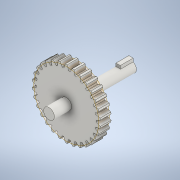
# Autodesk Inventor part: Spur Gear2
Saved by Autodesk Inventor 2021 (Build 250183000, 183)
## iProperties
Created: 2021-04-10
Part Number: Spur Gear2
Material: Steel
Document SubType Name: Modeling
Designer: Nabeel Azafer
Categories: <?xml version="1.0" encoding="UTF-16"?> <MemberInstance><Categories><FamilyTemplate><FamilyTemplateParameter ValueType="xs:double" Id="1" ObjectReferenceKey="da_z" ObjectType="kUserParameterObject"/><FamilyTemplateParameter ValueType="xs:double" Id="2" ObjectReferenceKey="da_b" ObjectType="kUserParameterObject"/><FamilyTemplateParameter ValueType="xs:double" Id="3" ObjectReferenceKey="da_beta" ObjectType="kUserParameterObject"/><FamilyTemplateParameter ValueType="xs:double" Id="4" ObjectReferenceKey="da_da" ObjectType="kUserParameterObject"/><FamilyTemplateParameter ValueType="xs:double" Id="5" ObjectReferenceKey="da_aw" ObjectType="kUserParameterObject"/><FamilyTemplateParameter ValueType="xs:string" Id="6" ObjectReferenceKey="EAIAABAAAACIAQAAAAAAAIAAAAAAAAAA" ObjectType="83910656" SubObjectId="SurfaceGeometry"/></FamilyTemplate><ParamToTemplateMap><ParamToTemplate CategoryParameter="//CategoryParameter[@InternalName='046C89C9-8512-4d59-83FE-43B91F4F132A']" TemplateParameter="1"/><ParamToTemplate CategoryParameter="//CategoryParameter[@InternalName='2552DF32-E462-4b46-AEBF-C6C7768E72AC']" TemplateParameter="2"/><ParamToTemplate CategoryParameter="//CategoryParameter[@InternalName='C9EE641D-15FC-4fae-A226-E94C4372FDD7']" TemplateParameter="3"/><ParamToTemplate><ParamToTemplate CategoryParameter="//CategoryParameter[@InternalName='00B6519A-459B-49c7-AD84-2E56D39A5744']" ConstantValue="0.000000"/></ParamToTemplate><ParamToTemplate><ParamToTemplate CategoryParameter="//CategoryParameter[@InternalName='04B31F0E-C7A6-4894-AA32-9629BEFACF47']" ConstantValue="0.800000"/></ParamToTemplate><ParamToTemplate><ParamToTemplate CategoryParameter="//CategoryParameter[@InternalName='43CBEC2E-7847-49e7-A936-2F7889FCB2D9']" ConstantValue="0.350000"/></ParamToTemplate><ParamToTemplate><ParamToTemplate CategoryParameter="//CategoryParameter[@InternalName='B1EFC894-105D-4ebd-86BF-FA20ED196853']" ConstantValue="0.500000"/></ParamToTemplate><ParamToTemplate><ParamToTemplate CategoryParameter="//CategoryParameter[@InternalName='51175063-3D10-4879-93E8-6246FE8B403D']" ConstantValue="2060000000.000000"/></ParamToTemplate><ParamToTemplate><ParamToTemplate CategoryParameter="//CategoryParameter[@InternalName='A3A52E27-4454-46a9-B0BD-C932399B70AF']" ConstantValue="0.300000"/></ParamToTemplate><ParamToTemplate><ParamToTemplate CategoryParameter="//CategoryParameter[@InternalName='91B76062-C214-41d9-B1B9-14D2AB99603D']" ConstantValue="0.100000"/></ParamToTemplate><ParamToTemplate><ParamToTemplate CategoryParameter="//CategoryParameter[@InternalName='374E806E-8B8A-4dda-A9AA-1039D6500AD2']" ConstantValue="10.000000"/></ParamToTemplate><ParamToTemplate><ParamToTemplate CategoryParameter="//CategoryParameter[@InternalName='2D373A89-B862-43d6-8D0B-0CBF12AB9F6C']" ConstantValue="0.349066"/></ParamToTemplate><ParamToTemplate CategoryParameter="//CategoryParameter[@InternalName='37777632-D6A2-4fac-9D53-DB8ACD95C989']" TemplateParameter="4"/><ParamToTemplate CategoryParameter="//CategoryParameter[@InternalName='FD1017F1-B727-4f7e-9707-0F86F1FF9423']" TemplateParameter="5"/><ParamToTemplate><ParamToTemplate CategoryParameter="//CategoryParameter[@InternalName='9E1B4470-B2D3-4ff1-B813-535BB4CDF51A']" ConstantValue="3520000.000000"/></ParamToTemplate><ParamToTemplate><ParamToTemplate CategoryParameter="//CategoryParameter[@InternalName='F8452263-BFF6-458c-9FB1-07C4B99E95CD']" ConstantValue="11400000.000000"/></ParamToTemplate><ParamToTemplate><ParamToTemplate CategoryParameter="//CategoryParameter[@InternalName='3E3BB259-FD49-497f-8171-6EBC954A3479']" ConstantValue="2.000000"/></ParamToTemplate><ParamToTemplate CategoryParameter="//CategoryParameter[@InternalName='27C3BAF2-7550-4e4b-AE2C-0DB134B7D9B7']" TemplateParameter="6"/></ParamToTemplateMap><Category DisplayName="Gear" InternalName="DC85795E-93AB-48d5-8EEE-5A27447B64BD" Mnemonic="Gear"><CategoryParameter DisplayName="z" InternalName="046C89C9-8512-4d59-83FE-43B91F4F132A" Mnemonic="z"/><CategoryParameter DisplayName="b" InternalName="2552DF32-E462-4b46-AEBF-C6C7768E72AC" Mnemonic="b"/><CategoryParameter DisplayName="||b|" InternalName="C9EE641D-15FC-4fae-A226-E94C4372FDD7" Mnemonic="beta"/><CategoryParameter DisplayName="x" InternalName="00B6519A-459B-49c7-AD84-2E56D39A5744" Mnemonic="x"/><CategoryParameter DisplayName="a*" InternalName="04B31F0E-C7A6-4894-AA32-9629BEFACF47" Mnemonic="a"/><CategoryParameter DisplayName="c*" InternalName="43CBEC2E-7847-49e7-A936-2F7889FCB2D9" Mnemonic="c"/><CategoryParameter DisplayName="r|.f|*" InternalName="B1EFC894-105D-4ebd-86BF-FA20ED196853" Mnemonic="rf"/><CategoryParameter DisplayName="E" InternalName="51175063-3D10-4879-93E8-6246FE8B403D" Mnemonic="E"/><CategoryParameter DisplayName="||m|" InternalName="A3A52E27-4454-46a9-B0BD-C932399B70AF" Mnemonic="mi"/><Category DisplayName="SpurGear" InternalName="26C5A22E-A91E-4dfd-A3B3-23CCAFAE1764" Mnemonic="SpurGear"><CategoryParameter DisplayName="m" InternalName="91B76062-C214-41d9-B1B9-14D2AB99603D" Mnemonic="m"/><CategoryParameter DisplayName="P" InternalName="374E806E-8B8A-4dda-A9AA-1039D6500AD2" Mnemonic="PP"/><CategoryParameter DisplayName="||a|" InternalName="2D373A89-B862-43d6-8D0B-0CBF12AB9F6C" Mnemonic="alpha"/><CategoryParameter DisplayName="d|.a|" InternalName="37777632-D6A2-4fac-9D53-DB8ACD95C989" Mnemonic="da"/><CategoryParameter DisplayName="a|.w|" InternalName="FD1017F1-B727-4f7e-9707-0F86F1FF9423" Mnemonic="aw"/><CategoryParameter DisplayName="||s||.Flim|" InternalName="9E1B4470-B2D3-4ff1-B813-535BB4CDF51A" Mnemonic="sFlim"/><CategoryParameter DisplayName="||s||.Hlim|" InternalName="F8452263-BFF6-458c-9FB1-07C4B99E95CD" Mnemonic="sHlim"/><CategoryParameter DisplayName="type" InternalName="3E3BB259-FD49-497f-8171-6EBC954A3479" Mnemonic="type"/><CategoryParameter DisplayName="PitchDiameter" InternalName="27C3BAF2-7550-4e4b-AE2C-0DB134B7D9B7" Mnemonic="IDS_PITCHDIAM"/></Category></Category></Categories></MemberInstance>
Density: 7.85 g/cm^3
Appearance: Steel
Mass: 43.2565 g
Surface Area: 28.3538 cm^2
Volume: 5.51038 cm^3
Author: Nabeel Azafer
Autodesk Inventor part; units mm, degrees
note: some values were not read from the file. Chosen so that the rebuilt part matches the saved one: direction of "Emboss1".
sketch "Sketch1" plane through (0, 0, 0) normal (0, 0, 1) x (1, 0, 0)
  circle A0 centre (0, 0) radius 15.8
  dimension "d0" = 31.6
  constraints: 1 centre point
  measures "d0" diameter of A0
extrude "Extrusion1" add sketch "Sketch1" along normal blind 5
ref_plane "Work Plane2" through (0, 0, 2.5) normal (0, 0, 1) x (1, 0, 0)
sketch "Sketch2" plane through (0, 0, 0) normal (0, 0, -1) x (-1, 0, 0)
  circle A0 centre (0, 0) radius 15.8 projected
  circle A1 centre (0, 0) radius 15
  dimension "d3" = 30
  constraints: 1 centre point, 1 coincident
  measures "d3" diameter of A1
surface extrude "Pitch Diameter" sketch "Sketch2" against normal through all shown yes curves A1
ref_plane "Work Plane8" through (0, 0, 0) normal (0.9945219, 0.1045285, 0) x (0, 0, 1)
ref_plane "Work Plane9" through (0, 0, 0) normal (1, 0, 0) x (0, 1, 0)
spur gear teeth "Spur Gear" teeth 30 pitch diameter 30 tip diameter 31.6 root diameter 27.7 face width 8 start plane through (0, 0, 0) normal (0, 0, -1) x (-1, 0, 0)
sketch "Sketch6" plane through (0, 0, 0) normal (0, 0, -1) x (-1, 0, 0)
  circle A0 centre (0, 0) radius 2.5
  dimension "d68" = 5
  constraints: 1 centre point, 1 coincident
  measures "d68" diameter of A0
extrude "Extrusion4" add sketch "Sketch6" along normal blind 25
sketch "Sketch7" plane through (0, 0, -25) normal (0, 0, -1) x (-1, 0, 0)
  circle A0 centre (0, 0) radius 2.5 projected
  line L0 (-1, 2.2913) -> (1, 2.2913)
  line L1 (1, 2.2913) -> (1, 3.7913)
  line L2 (1, 3.7913) -> (-1, 3.7913)
  line L3 (-1, 3.7913) -> (-1, 2.2913)
  dimension "d75" = 2
  dimension "d76" = 1.5
  constraints: 8 end point, 2 parallel, 1 horizontal, 1 perpendicular, 2 other
  measures "d75" distance of L2.end L1.end
  measures "d76" distance of L1.end L0.end
extrude "Extrusion5" add sketch "Sketch7" against normal blind 6 contours L0 A0 | A0 L3 L2 L1 picked at (-0.1703, 2.3433)
sketch "Sketch8" plane through (0, 0, 5) normal (0, 0, 1) x (1, 0, 0)
  circle A0 centre (0, 0) radius 2.5
  dimension "d79" = 5
  constraints: 1 centre point, 1 coincident
  measures "d79" diameter of A0
extrude "Extrusion6" add sketch "Sketch8" along normal blind 8
sketch "Sketch9" plane through (0, 0, 0) normal (0, 0, -1) x (-1, 0, 0)
  line L0 (-6.4513, 9.2943) -> (6.8887, 9.2943) construction
  line L1 (6.8887, 9.2943) -> (6.8887, 2.6243) construction
  line L2 (6.8887, 2.6243) -> (-6.4513, 2.6243) construction
  line L3 (-6.4513, 2.6243) -> (-6.4513, 9.2943) construction
  spline S0 degree 2 poles (-5.4108, 7.2132) (-5.6231, 7.2132) (-5.9748, 7.3429) (-6.1012, 7.4742) knots 0 0 0 1 2 2 2
  spline S1 degree 2 poles (-6.1012, 7.4742) (-6.2277, 7.6071) (-6.3622, 7.9993) (-6.3622, 8.2538) knots 0 0 0 1 2 2 2
  spline S2 degree 2 poles (-6.3622, 8.2538) (-6.3622, 8.4953) (-6.226, 8.8777) (-6.0996, 9.0139) knots 0 0 0 1 2 2 2
  spline S3 degree 2 poles (-6.0996, 9.0139) (-5.9781, 9.1452) (-5.6215, 9.2878) (-5.4092, 9.2878) knots 0 0 0 1 2 2 2
  spline S4 degree 2 poles (-5.4092, 9.2878) (-5.3071, 9.2878) (-5.1223, 9.2586) (-5.038, 9.2327) knots 0 0 0 1 2 2 2
  spline S5 degree 2 poles (-5.038, 9.2327) (-4.97, 9.2132) (-4.8046, 9.1419) (-4.7544, 9.116) knots 0 0 0 1 2 2 2
  line L4 (-4.7544, 9.116) -> (-4.7544, 8.7951)
  line L5 (-4.7544, 8.7951) -> (-4.7771, 8.7951)
  spline S6 degree 2 poles (-4.7771, 8.7951) (-4.8273, 8.8389) (-4.9327, 8.9183) (-5.0299, 8.9636) knots 0 0 0 1 2 2 2
  spline S7 degree 2 poles (-5.0299, 8.9636) (-5.111, 9.0042) (-5.32, 9.0577) (-5.44, 9.0577) knots 0 0 0 1 2 2 2
  spline S8 degree 2 poles (-5.44, 9.0577) (-5.7285, 9.0577) (-6.085, 8.6233) (-6.085, 8.2619) knots 0 0 0 1 2 2 2
  spline S9 degree 2 poles (-6.085, 8.2619) (-6.085, 8.0609) (-5.991, 7.7594) (-5.9019, 7.6557) knots 0 0 0 1 2 2 2
  spline S10 degree 2 poles (-5.9019, 7.6557) (-5.816, 7.552) (-5.5729, 7.4434) (-5.4205, 7.4434) knots 0 0 0 1 2 2 2
  spline S11 degree 2 poles (-5.4205, 7.4434) (-5.3087, 7.4434) (-5.085, 7.4758) (-5.0089, 7.5082) knots 0 0 0 1 2 2 2
  line L6 (-5.0089, 7.5082) -> (-5.0089, 8.0252)
  line L7 (-5.0089, 8.0252) -> (-5.4724, 8.0252)
  line L8 (-5.4724, 8.0252) -> (-5.4724, 8.2586)
  line L9 (-5.4724, 8.2586) -> (-4.7463, 8.2586)
  line L10 (-4.7463, 8.2586) -> (-4.7463, 7.385)
  spline S12 degree 2 poles (-4.7463, 7.385) (-4.7965, 7.3624) (-4.9683, 7.2927) (-5.0413, 7.2716) knots 0 0 0 1 2 2 2
  spline S13 degree 2 poles (-5.0413, 7.2716) (-5.1401, 7.2424) (-5.299, 7.2132) (-5.4108, 7.2132) knots 0 0 0 1 2 2 2
  spline S14 degree 2 poles (-3.7803, 7.2181) (-4.1401, 7.2181) (-4.5356, 7.6217) (-4.5356, 7.9944) knots 0 0 0 1 2 2 2
  spline S15 degree 2 poles (-4.5356, 7.9944) (-4.5356, 8.3607) (-4.1515, 8.7951) (-3.8419, 8.7951) knots 0 0 0 1 2 2 2
  spline S16 degree 2 poles (-3.8419, 8.7951) (-3.7025, 8.7951) (-3.487, 8.7141) (-3.4076, 8.6282) knots 0 0 0 1 2 2 2
  spline S17 degree 2 poles (-3.4076, 8.6282) (-3.3265, 8.5423) (-3.2406, 8.2943) (-3.2406, 8.1144) knots 0 0 0 1 2 2 2
  line L11 (-3.2406, 8.1144) -> (-3.2406, 7.9766)
  line L12 (-3.2406, 7.9766) -> (-4.2795, 7.9766)
  spline S18 degree 2 poles (-4.2795, 7.9766) (-4.2795, 7.7157) (-4.017, 7.4385) (-3.7836, 7.4385) knots 0 0 0 1 2 2 2
  spline S19 degree 2 poles (-3.7836, 7.4385) (-3.7009, 7.4385) (-3.5405, 7.4758) (-3.4756, 7.505) knots 0 0 0 1 2 2 2
  spline S20 degree 2 poles (-3.4756, 7.505) (-3.4076, 7.5374) (-3.3136, 7.5941) (-3.2828, 7.6201) knots 0 0 0 1 2 2 2
  line L13 (-3.2828, 7.6201) -> (-3.2682, 7.6201)
  line L14 (-3.2682, 7.6201) -> (-3.2682, 7.3445)
  spline S21 degree 2 poles (-3.2682, 7.3445) (-3.3119, 7.3267) (-3.4448, 7.2748) (-3.4967, 7.2602) knots 0 0 0 1 2 2 2
  spline S22 degree 2 poles (-3.4967, 7.2602) (-3.5696, 7.2392) (-3.6896, 7.2181) (-3.7803, 7.2181) knots 0 0 0 1 2 2 2
  spline S23 degree 2 poles (-3.487, 8.1695) (-3.4902, 8.2716) (-3.5324, 8.4207) (-3.5729, 8.4709) knots 0 0 0 1 2 2 2
  spline S24 degree 2 poles (-3.5729, 8.4709) (-3.6166, 8.5277) (-3.7544, 8.5876) (-3.8565, 8.5876) knots 0 0 0 1 2 2 2
  spline S25 degree 2 poles (-3.8565, 8.5876) (-3.957, 8.5876) (-4.098, 8.5277) (-4.1563, 8.4693) knots 0 0 0 1 2 2 2
  spline S26 degree 2 poles (-4.1563, 8.4693) (-4.2131, 8.4094) (-4.2714, 8.2651) (-4.2795, 8.1695) knots 0 0 0 1 2 2 2
  line L15 (-4.2795, 8.1695) -> (-3.487, 8.1695)
  spline S27 degree 2 poles (-2.1482, 7.411) (-2.179, 7.3883) (-2.2828, 7.3072) (-2.3314, 7.2829) knots 0 0 0 1 2 2 2
  spline S28 degree 2 poles (-2.3314, 7.2829) (-2.3978, 7.2473) (-2.5226, 7.21) (-2.6361, 7.21) knots 0 0 0 1 2 2 2
  spline S29 degree 2 poles (-2.6361, 7.21) (-2.7285, 7.21) (-2.8954, 7.2797) (-2.9586, 7.3429) knots 0 0 0 1 2 2 2
  spline S30 degree 2 poles (-2.9586, 7.3429) (-3.0186, 7.4045) (-3.0915, 7.586) (-3.0915, 7.6865) knots 0 0 0 1 2 2 2
  spline S31 degree 2 poles (-3.0915, 7.6865) (-3.0915, 7.8421) (-2.9602, 8.0625) (-2.8176, 8.1257) knots 0 0 0 1 2 2 2
  spline S32 degree 2 poles (-2.8176, 8.1257) (-2.6912, 8.1841) (-2.3476, 8.2278) (-2.1482, 8.2392) knots 0 0 0 1 2 2 2
  line L16 (-2.1482, 8.2392) -> (-2.1482, 8.2878)
  spline S33 degree 2 poles (-2.1482, 8.2878) (-2.1482, 8.3753) (-2.2017, 8.4839) (-2.2504, 8.5147) knots 0 0 0 1 2 2 2
  spline S34 degree 2 poles (-2.2504, 8.5147) (-2.299, 8.5455) (-2.4384, 8.5649) (-2.5129, 8.5649) knots 0 0 0 1 2 2 2
  spline S35 degree 2 poles (-2.5129, 8.5649) (-2.6004, 8.5649) (-2.8371, 8.5131) (-2.9554, 8.4628) knots 0 0 0 1 2 2 2
  line L17 (-2.9554, 8.4628) -> (-2.97, 8.4628)
  line L18 (-2.97, 8.4628) -> (-2.97, 8.7205)
  spline S36 degree 2 poles (-2.97, 8.7205) (-2.9003, 8.74) (-2.6393, 8.7886) (-2.5113, 8.7886) knots 0 0 0 1 2 2 2
  spline S37 degree 2 poles (-2.5113, 8.7886) (-2.3557, 8.7886) (-2.1434, 8.74) (-2.0591, 8.6768) knots 0 0 0 1 2 2 2
  spline S38 degree 2 poles (-2.0591, 8.6768) (-1.9764, 8.6152) (-1.8954, 8.4191) (-1.8954, 8.2781) knots 0 0 0 1 2 2 2
  line L19 (-1.8954, 8.2781) -> (-1.8954, 7.2521)
  line L20 (-1.8954, 7.2521) -> (-2.1482, 7.2521)
  line L21 (-2.1482, 7.2521) -> (-2.1482, 7.411)
  line L22 (-2.1482, 7.6217) -> (-2.1482, 8.0382)
  spline S39 degree 2 poles (-2.1482, 8.0382) (-2.239, 8.0301) (-2.5129, 8.0025) (-2.5988, 7.9766) knots 0 0 0 1 2 2 2
  spline S40 degree 2 poles (-2.5988, 7.9766) (-2.6993, 7.9458) (-2.8306, 7.8178) (-2.8306, 7.7043) knots 0 0 0 1 2 2 2
  spline S41 degree 2 poles (-2.8306, 7.7043) (-2.8306, 7.5747) (-2.6847, 7.4434) (-2.5453, 7.4434) knots 0 0 0 1 2 2 2
  spline S42 degree 2 poles (-2.5453, 7.4434) (-2.427, 7.4434) (-2.2325, 7.5455) (-2.1482, 7.6217) knots 0 0 0 1 2 2 2
  line L23 (-0.7447, 8.4823) -> (-0.7576, 8.4823)
  spline S43 degree 2 poles (-0.7576, 8.4823) (-0.7868, 8.4904) (-0.85, 8.4936) (-0.8938, 8.4936) knots 0 0 0 1 2 2 2
  spline S44 degree 2 poles (-0.8938, 8.4936) (-0.9959, 8.4936) (-1.1969, 8.4045) (-1.2876, 8.317) knots 0 0 0 1 2 2 2
  line L24 (-1.2876, 8.317) -> (-1.2876, 7.2521)
  line L25 (-1.2876, 7.2521) -> (-1.5405, 7.2521)
  line L26 (-1.5405, 7.2521) -> (-1.5405, 8.753)
  line L27 (-1.5405, 8.753) -> (-1.2876, 8.753)
  line L28 (-1.2876, 8.753) -> (-1.2876, 8.5293)
  spline S45 degree 2 poles (-1.2876, 8.5293) (-1.1499, 8.6525) (-0.944, 8.753) (-0.8468, 8.753) knots 0 0 0 1 2 2 2
  spline S46 degree 2 poles (-0.8468, 8.753) (-0.8079, 8.753) (-0.769, 8.7497) (-0.7447, 8.7448) knots 0 0 0 1 2 2 2
  line L29 (-0.7447, 8.7448) -> (-0.7447, 8.4823)
  spline S47 degree 2 poles (0.8129, 9.0625) (0.7399, 9.0625) (0.5957, 9.0269) (0.526, 8.9993) knots 0 0 0 1 2 2 2
  spline S48 degree 2 poles (0.526, 8.9993) (0.4612, 8.9718) (0.3655, 8.9134) (0.3283, 8.8875) knots 0 0 0 1 2 2 2
  line L30 (0.3283, 8.8875) -> (0.312, 8.8875)
  line L31 (0.312, 8.8875) -> (0.312, 9.1711)
  spline S49 degree 2 poles (0.312, 9.1711) (0.3996, 9.2181) (0.6994, 9.2943) (0.8339, 9.2943) knots 0 0 0 1 2 2 2
  spline S50 degree 2 poles (0.8339, 9.2943) (0.9701, 9.2943) (1.1727, 9.2392) (1.2553, 9.1808) knots 0 0 0 1 2 2 2
  spline S51 degree 2 poles (1.2553, 9.1808) (1.3428, 9.1176) (1.4336, 8.9345) (1.4336, 8.8113) knots 0 0 0 1 2 2 2
  spline S52 degree 2 poles (1.4336, 8.8113) (1.4336, 8.646) (1.2164, 8.3964) (1.0641, 8.364) knots 0 0 0 1 2 2 2
  line L32 (1.0641, 8.364) -> (1.0641, 8.3445)
  spline S53 degree 2 poles (1.0641, 8.3445) (1.1273, 8.3316) (1.2715, 8.2732) (1.3331, 8.2149) knots 0 0 0 1 2 2 2
  spline S54 degree 2 poles (1.3331, 8.2149) (1.3947, 8.1581) (1.4725, 7.9766) (1.4725, 7.8453) knots 0 0 0 1 2 2 2
  spline S55 degree 2 poles (1.4725, 7.8453) (1.4725, 7.7108) (1.3801, 7.4823) (1.2958, 7.3948) knots 0 0 0 1 2 2 2
  spline S56 degree 2 poles (1.2958, 7.3948) (1.2083, 7.304) (0.9603, 7.21) (0.8031, 7.21) knots 0 0 0 1 2 2 2
  spline S57 degree 2 poles (0.8031, 7.21) (0.6524, 7.21) (0.3574, 7.2829) (0.2569, 7.3332) knots 0 0 0 1 2 2 2
  line L33 (0.2569, 7.3332) -> (0.2569, 7.6168)
  line L34 (0.2569, 7.6168) -> (0.2764, 7.6168)
  spline S58 degree 2 poles (0.2764, 7.6168) (0.3607, 7.5552) (0.6459, 7.4418) (0.7869, 7.4418) knots 0 0 0 1 2 2 2
  spline S59 degree 2 poles (0.7869, 7.4418) (0.8696, 7.4418) (1.0349, 7.4936) (1.09, 7.5536) knots 0 0 0 1 2 2 2
  spline S60 degree 2 poles (1.09, 7.5536) (1.1435, 7.6136) (1.2002, 7.7562) (1.2002, 7.8648) knots 0 0 0 1 2 2 2
  spline S61 degree 2 poles (1.2002, 7.8648) (1.2002, 7.9734) (1.137, 8.1144) (1.0803, 8.1549) knots 0 0 0 1 2 2 2
  spline S62 degree 2 poles (1.0803, 8.1549) (1.0236, 8.1954) (0.8696, 8.2262) (0.7788, 8.2262) knots 0 0 0 1 2 2 2
  line L35 (0.7788, 8.2262) -> (0.6654, 8.2262)
  line L36 (0.6654, 8.2262) -> (0.6654, 8.4483)
  line L37 (0.6654, 8.4483) -> (0.7545, 8.4483)
  spline S63 degree 2 poles (0.7545, 8.4483) (0.9344, 8.4483) (1.1613, 8.6201) (1.1613, 8.7837) knots 0 0 0 1 2 2 2
  spline S64 degree 2 poles (1.1613, 8.7837) (1.1613, 8.8599) (1.103, 8.9685) (1.056, 9.0009) knots 0 0 0 1 2 2 2
  spline S65 degree 2 poles (1.056, 9.0009) (1.0057, 9.035) (0.8825, 9.0625) (0.8129, 9.0625) knots 0 0 0 1 2 2 2
  spline S66 degree 2 poles (3.0187, 8.2521) (3.0187, 7.7141) (2.7059, 7.21) (2.3801, 7.21) knots 0 0 0 1 2 2 2
  spline S67 degree 2 poles (2.3801, 7.21) (2.0495, 7.21) (1.7399, 7.7238) (1.7399, 8.2505) knots 0 0 0 1 2 2 2
  spline S68 degree 2 poles (1.7399, 8.2505) (1.7399, 8.7918) (2.0527, 9.2927) (2.3801, 9.2927) knots 0 0 0 1 2 2 2
  spline S69 degree 2 poles (2.3801, 9.2927) (2.7091, 9.2927) (3.0187, 8.774) (3.0187, 8.2521) knots 0 0 0 1 2 2 2
  spline S70 degree 2 poles (2.6751, 7.6427) (2.714, 7.7416) (2.7464, 8.0463) (2.7464, 8.2521) knots 0 0 0 1 2 2 2
  spline S71 degree 2 poles (2.7464, 8.2521) (2.7464, 8.458) (2.714, 8.7611) (2.6735, 8.8632) knots 0 0 0 1 2 2 2
  spline S72 degree 2 poles (2.6735, 8.8632) (2.633, 8.9653) (2.4919, 9.0706) (2.3801, 9.0706) knots 0 0 0 1 2 2 2
  spline S73 degree 2 poles (2.3801, 9.0706) (2.2683, 9.0706) (2.124, 8.9653) (2.0819, 8.8599) knots 0 0 0 1 2 2 2
  spline S74 degree 2 poles (2.0819, 8.8599) (2.0414, 8.7578) (2.0122, 8.4466) (2.0122, 8.2505) knots 0 0 0 1 2 2 2
  spline S75 degree 2 poles (2.0122, 8.2505) (2.0122, 8.0398) (2.0381, 7.7578) (2.0803, 7.6476) knots 0 0 0 1 2 2 2
  spline S76 degree 2 poles (2.0803, 7.6476) (2.1192, 7.5439) (2.2634, 7.432) (2.3801, 7.432) knots 0 0 0 1 2 2 2
  spline S77 degree 2 poles (2.3801, 7.432) (2.4903, 7.432) (2.6346, 7.5374) (2.6751, 7.6427) knots 0 0 0 1 2 2 2
  line L38 (3.9749, 7.2521) -> (4.6492, 9.2521)
  line L39 (4.6492, 9.2521) -> (4.9766, 9.2521)
  line L40 (4.9766, 9.2521) -> (5.6508, 7.2521)
  line L41 (5.6508, 7.2521) -> (5.3704, 7.2521)
  line L42 (5.3704, 7.2521) -> (5.1889, 7.8113)
  line L43 (5.1889, 7.8113) -> (4.4255, 7.8113)
  line L44 (4.4255, 7.8113) -> (4.244, 7.2521)
  line L45 (4.244, 7.2521) -> (3.9749, 7.2521)
  line L46 (5.1159, 8.0382) -> (4.8064, 8.9799)
  line L47 (4.8064, 8.9799) -> (4.4984, 8.0382)
  line L48 (4.4984, 8.0382) -> (5.1159, 8.0382)
  point P0 (0, 0)
  constraints: 2 other
emboss "Emboss1" sketch "Sketch9" operation cut depth 1 direction (0, 0, 1)
equation "\"d0\" = da_da"
equation "\"d3\" = da_d"
equation "\"d16\" = da_aw"
equation "\"d43\" = da_aw"
equation "\"d46\" = da_aw"
equation "\"da_da\" = 31.6"
equation "\"da_d\" = 30"
equation "\"da_aw\" = 22.5"
body "Solid1"
body "Srf1"
